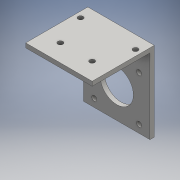
# Autodesk Inventor part: 电机座2
Saved by Autodesk Inventor 2016 (Build 200138000, 138)
## iProperties
Created: 2019-04-02
Part Number: 电机座2
Material: 常规
Document SubType Name: Modeling
Designer: oldboy
Density: 1 g/cm^3
Appearance: 默认
Author: oldboy
Autodesk Inventor part; units mm, degrees
ref_plane "YZ Plane" through (0, 0, 0) normal (1, 0, 0) x (0, 1, 0)
ref_plane "XZ Plane" through (0, 0, 0) normal (0, 1, 0) x (-1, 0, 0)
ref_plane "XY Plane" through (0, 0, 0) normal (0, 0, 1) x (1, 0, 0)
sketch "草图2" plane through (0, 0, 0) normal (0, 1, 0) x (-1, 0, 0)
  line L0 (-21, 21) -> (21, 21)
  line L1 (21, 21) -> (21, -21)
  line L2 (21, -21) -> (-21, -21)
  line L3 (-21, -21) -> (-21, 21)
  line L4 (-21, 21) -> (21, -21) construction
  line L5 (21, 21) -> (-21, -21) construction
  point P0 (0, 0)
  dimension "d3" = 42
  dimension "d4" = 42
  constraints: 12 end point, 2 midpoint, 2 parallel, 1 horizontal, 1 perpendicular
  measures "d3" distance between parallel lines of L3 L1
  measures "d4" distance between parallel lines of L2 L0
extrude "拉伸2" add sketch "草图2" along normal blind 3
sketch "草图3" plane through (-21, 0, 21) normal (0, 0, 1) x (1, 0, 0)
  line L0 (0, 3) -> (42, 3) projected
  line L1 (0, 3) -> (42, 3)
  line L2 (42, 3) -> (42, -40)
  line L3 (42, -40) -> (0, -40)
  line L4 (0, -40) -> (0, 3)
  point P0 (21, 0)
  dimension "d7" = 43
  constraints: 8 end point, 2 parallel, 1 horizontal, 1 perpendicular
  measures "d7" distance between parallel lines of L3 L0
extrude "拉伸3" add sketch "草图3" along normal blind 3
sketch "草图7" plane through (0, 0, 0) normal (0, -1, 0) x (1, 0, 0)
  circle A0 centre (0, 0) radius 11.5
  circle A1 centre (-15.5, 15.5) radius 1.75
  circle A2 centre (-15.5, -15.5) radius 1.75
  circle A3 centre (15.5, -15.5) radius 1.75
  circle A4 centre (15.5, 15.5) radius 1.75
  dimension "d17" = 23
  dimension "d18" = 3.5
  dimension "d19" = 15.5
  dimension "d20" = 15.5
  dimension "d21" = 15.5
  dimension "d22" = 15.5
  constraints: 5 centre point, 3 equal radius, 2 horizontal alignment, 2 vertical alignment, 1 coincident
  measures "d17" diameter of A0
  measures "d18" diameter of A2
  measures "d19" horizontal distance of point (0, 0) A2.centre
  measures "d20" horizontal distance of point (0, 0) A2.centre
  measures "d21" horizontal distance of point (0, 0) A1.centre
  measures "d22" horizontal distance of point (0, 0) A3.centre
extrude "拉伸6" cut sketch "草图7" against normal blind 3
sketch "草图9" plane through (-21, 0, 21) normal (0, 0, -1) x (-1, 0, 0)
  circle A0 centre (-40, -6) radius 1.75
  line L0 (0, 0) -> (-42, 0) projected
  line L1 (-42, 3) -> (0, 3) projected
  line L2 (-21, 0) -> (-21, -40) construction
  line L3 (0, -40) -> (-42, -40) projected
  circle A1 centre (-2, -6) radius 1.75
  circle A2 centre (-32, -28) radius 1.75
  circle A3 centre (-10, -28) radius 1.75
  dimension "d32" = 3.5
  dimension "d34" = 9
  dimension "d35" = 19
  dimension "d36" = 3.5
  dimension "d37" = 11
  dimension "d38" = 22
  constraints: 4 centre point, 2 end point, 2 symmetric about line, 1 midpoint, 2 other
  measures "d32" diameter of A0
  measures "d34" distance from line of A0.centre L1
  measures "d35" distance from line of L2 A0.centre
  measures "d36" diameter of A2
  measures "d37" distance from line of L2 A2.centre
  measures "d38" vertical distance of A0.centre A2.centre
extrude "拉伸8" cut sketch "草图9" against normal blind 10
sketch "草图10" plane through (21, 0, -21) normal (1, 0, 0) x (0, 0, -1)
  line L0 (0, 0) -> (-42, 0) projected
  line L1 (0, 0) -> (0, 3) projected
  line L2 (0, 3) -> (-45, 3) projected
  line L3 (-45, -40) -> (-45, 3) projected
  line L4 (-42, -40) -> (-45, -40) projected
  line L5 (-42, -40) -> (-42, 0) projected
  point P0 (-21, 0)
extrude "拉伸9" add sketch "草图10" along normal blind 2
sketch "草图11" plane through (-21, 0, -21) normal (-1, 0, 0) x (0, 0, 1)
  line L0 (42, 0) -> (0, 0) projected
  line L1 (42, 0) -> (42, -40) projected
  line L2 (42, -40) -> (45, -40) projected
  line L3 (45, 3) -> (45, -40) projected
  line L4 (0, 3) -> (45, 3) projected
  line L5 (0, 0) -> (0, 3) projected
  point P0 (21, 0)
extrude "拉伸10" add sketch "草图11" along normal blind 2
sketch "草图12" plane through (-21, 0, 24) normal (0, 0, 1) x (1, 0, 0)
  circle A0 centre (32, -28) radius 1.75 projected
  circle A1 centre (40, -6) radius 1.75 projected
  circle A2 centre (2, -6) radius 1.75 projected
  circle A3 centre (10, -28) radius 1.75 projected
  line L0 (44, -40) -> (-2, -40) projected
  line L1 (44, 3) -> (44, -40) projected
  line L2 (-2, 3) -> (44, 3) projected
  line L3 (-2, -40) -> (-2, 3) projected
  point P0 (21, 0)
extrude "拉伸11" add sketch "草图12" along normal blind 10
sketch "草图13" plane through (-21, 0, 21) normal (0, 0, -1) x (-1, 0, 0)
  circle A0 centre (-32, -28) radius 1.75 projected
  circle A1 centre (-40, -6) radius 1.75 projected
  circle A2 centre (-2, -6) radius 1.75 projected
  circle A3 centre (-10, -28) radius 1.75 projected
  line L0 (-44, 0) -> (2, 0) projected
  line L1 (-44, -40) -> (-44, 0) projected
  line L2 (-44, -40) -> (2, -40) projected
  line L3 (2, 0) -> (2, -40) projected
  point P0 (-21, 0)
extrude "拉伸12" cut sketch "草图13" against normal blind 10
